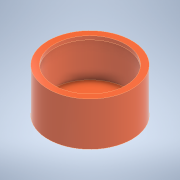
# Autodesk Inventor part: box
Saved by Autodesk Inventor 2022.2 (Build 262287000, 287)
## iProperties
Created: 2022-02-21
Part Number: box
Material: Steel, Carbon
Document SubType Name: Sheet Metal
Designer: PRASHANTH
Density: 7.85 g/cm^3
Sheet Metal Rule: Default_mm
Appearance: Smooth - Light Orange
Author: PRASHANTH
Autodesk Inventor part; units mm, degrees
ref_plane "YZ Plane" through (0, 0, 0) normal (1, 0, 0) x (0, 1, 0)
ref_plane "XZ Plane" through (0, 0, 0) normal (0, 1, 0) x (-1, 0, 0)
ref_plane "XY Plane" through (0, 0, 0) normal (0, 0, 1) x (1, 0, 0)
sketch "Sketch1" plane through (0, 0, 0) normal (0, 0, 1) x (1, 0, 0)
  line L0 (-6.9059, 7.4416) -> (-6.9059, -42.5584)
  line L1 (-6.9059, -42.5584) -> (45.659, -42.5584)
  line L2 (45.659, -42.5584) -> (-4.341, -42.5584)
  line L3 (-6.9059, 7.4416) -> (45.659, 7.4416)
  line L4 (45.659, 7.4416) -> (45.659, -42.5584)
  point P0 (0, 0)
  dimension "d0" = 50
  dimension "d1" = 50
  constraints: 10 end point, 2 perpendicular, 1 point on line, 1 vertical
  measures "d0" distance of L0.start L0.end
  measures "d1" distance of L1.end L2.end
revolve "Revolution1" add sketch "Sketch1" angle 360 about axis through (45.659, 7.4416, 0) along (0, -1, 0)
shell "Shell1" thickness 5 outward yes removed faces 0
sketch "Sketch2" plane through (45.659, 12.4416, 0) normal (0, 1, 0) x (1, 0, 0)
  circle A0 centre (0, 0) radius 49.1631
  point P0 (-45.659, 0)
  constraints: 1 centre point
extrude "Extrusion1" cut sketch "Sketch2" against normal blind 45
equation "\"BendRadius\" = Thickness"
equation "\"BendReliefWidth\" = Thickness"
equation "\"BendReliefDepth\" = 0.5 * Thickness"
equation "\"CornerReliefSize\" = 4 * Thickness"
equation "\"MinimumRemnant\" = 2 * Thickness"
equation "\"TransitionRadius\" = BendRadius"
equation "\"JacobiRadiusSize\" = BendRadius"
equation "\"GapSize\" = Thickness"
equation "\"Thickness\" = 0.5"
body "Solid1"
